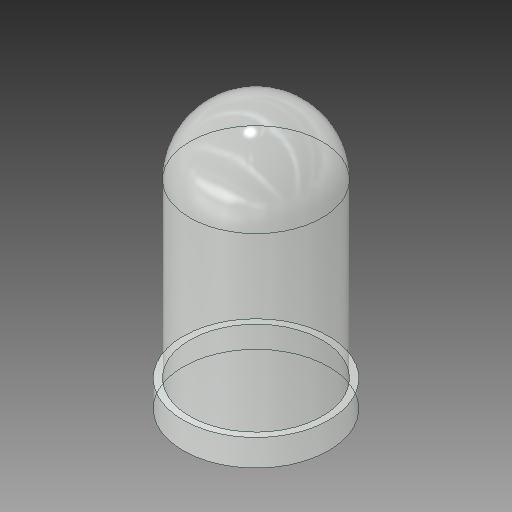
# Autodesk Inventor part: Head
Saved by Autodesk Inventor 2019.3 (Build 233278000, 278)
## iProperties
Created: 2019-01-06
Part Number: Head
Material: Glas
Document SubType Name: Modeling
Designer: Jonas
Density: 2.18 g/cm^3
Appearance: Klar
Author: Jonas
Autodesk Inventor part; units mm, degrees
ref_plane "YZ Plane" through (0, 0, 0) normal (1, 0, 0) x (0, 1, 0)
ref_plane "XZ Plane" through (0, 0, 0) normal (0, 1, 0) x (-1, 0, 0)
ref_plane "XY Plane" through (0, 0, 0) normal (0, 0, 1) x (1, 0, 0)
sketch "Skizze2" plane through (0, 0, 0) normal (0, 1, 0) x (-1, 0, 0)
  circle A0 centre (0, 0) radius 2.5
  circle A1 centre (0, 0) radius 2.75
  dimension "d0" = 5
  dimension "d4" = 0.25
  constraints: 2 centre point, 1 coincident
  measures "d0" diameter of A0
  measures "d4" radial gap between concentric circles of A1 A0
extrude "Extrusion1" add sketch "Skizze2" along normal blind 9 contours A0
fillet "Rundung1" radius 2.5 1 edges at (2.5, 9, 0)
extrude "Extrusion2" add sketch "Skizze2" against normal blind 1 contours A0 | A1
